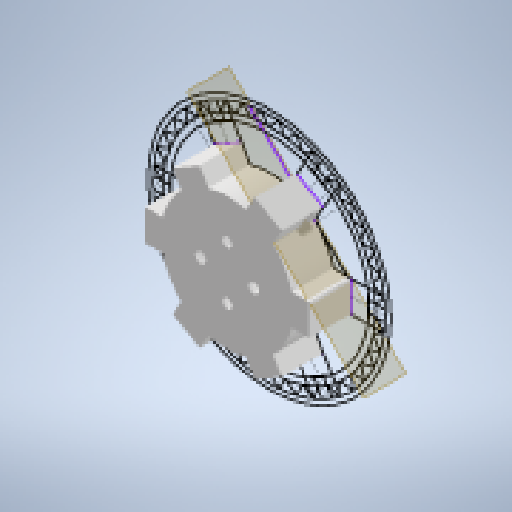
# Autodesk Inventor part: inside_part_wheel
Saved by Autodesk Inventor 2023 (Build 270158000, 158)
## iProperties
Created: 2026-02-22
Part Number: inside_part_wheel
Material: Типовые
Document SubType Name: Modeling
Designer: garin
Density: 1 g/cm^3
Appearance: По умолчанию
Author: garin
Autodesk Inventor part; units mm, degrees
note: some values were not read from the file. Chosen so that the rebuilt part matches the saved one: second side of "Выдавливание1".
ref_plane "YZ Plane" through (0, 0, 0) normal (1, 0, 0) x (0, 1, 0)
sketch "Эскиз1" plane through (0, 0, 0) normal (0, 0, 1) x (1, 0, 0)
  line L0 (0, 0) -> (34.5691, 5.4752) construction
  line L1 (0, 0) -> (35, 0) construction
  line L2 (0, 0) -> (34.5691, -5.4752) construction
  circle A0 centre (0, 0) radius 11.25
  circle A1 centre (0, 0) radius 15
  circle A2 centre (0, 0) radius 20
  circle A3 centre (0, 0) radius 30.0525
  circle A4 centre (0, 0) radius 32.0038
  circle A5 centre (0, 0) radius 35
  line L3 (0, 0) -> (17.5, -30.3109) construction
  circle A6 centre (0, -8) radius 1.5
  circle A7 centre (-8, 0) radius 1.5
  line L4 (0, 0) -> (-35, 0) construction
  line L5 (-29.6307, -4.693) -> (-19.4416, -4.693) construction
  line L6 (-29.6307, -4.693) -> (-19.4416, -4.693)
  line L7 (-29.6839, -4.693) -> (-29.6839, 4.693)
  line L8 (-19.4416, 4.693) -> (-34.6839, 4.693) construction
  line L9 (-19.4416, -4.693) -> (-34.6839, -4.693) construction
  line L10 (10.751, 28.0074) -> (5.6565, 19.1834) construction
  line L11 (5.6565, 19.1834) -> (13.2777, 32.3837) construction
  line L12 (-5.6565, 19.1834) -> (-13.2777, 32.3837) construction
  circle A8 centre (0, 8) radius 1.5
  line L13 (0, 0) -> (-17.5, 30.3109) construction
  line L14 (-5.6565, 19.1834) -> (-13.2777, 32.3837)
  line L15 (0, 0) -> (17.5, 30.3109) construction
  line L16 (0, 0) -> (-17.5, -30.3109) construction
  line L17 (5.6565, 19.1834) -> (13.2777, 32.3837)
  line L18 (13.3758, 26.5536) -> (16.0133, 31.1219)
  line L19 (16.3082, 24.8605) -> (18.9457, 29.4289)
  line L20 (18.9457, 29.4289) -> (17.4457, 26.8308) construction
  line L21 (29.6307, 4.693) -> (19.4416, 4.693)
  line L22 (18.8796, -23.3144) -> (13.7851, -14.4904) construction
  line L23 (13.7851, -14.4904) -> (21.4063, -27.6907) construction
  line L24 (29.6839, 4.693) -> (29.6839, 1.693)
  line L25 (29.6839, 4.693) -> (29.6839, -4.693)
  line L26 (29.6839, -4.693) -> (29.6839, -1.693) construction
  circle A9 centre (8, 0) radius 1.5
  line L27 (-18.8796, 23.3144) -> (-13.7851, 14.4904) construction
  line L28 (-13.7851, 14.4904) -> (-21.4063, 27.6907) construction
  line L29 (-18.8796, 23.3144) -> (-13.7851, 14.4904)
  line L30 (-13.7851, 14.4904) -> (-21.4063, 27.6907)
  line L31 (-18.9063, 23.3605) -> (-10.7777, 28.0536)
  line L32 (-16.3082, 24.8605) -> (-18.9457, 29.4289)
  line L33 (-13.3758, 26.5536) -> (-16.0133, 31.1219)
  line L34 (-13.7851, -14.4904) -> (-21.4063, -27.6907) construction
  line L35 (-10.751, -28.0074) -> (-5.6565, -19.1834) construction
  line L36 (-13.7851, -14.4904) -> (-21.4063, -27.6907)
  line L37 (-10.751, -28.0074) -> (-5.6565, -19.1834)
  line L38 (13.7851, 14.4904) -> (21.4063, 27.6907) construction
  line L39 (21.4063, 27.6907) -> (20.1674, 25.5449) construction
  line L40 (10.7777, 28.0536) -> (18.9063, 23.3605)
  line L41 (13.7851, 14.4904) -> (21.4063, 27.6907)
  line L42 (10.751, 28.0074) -> (5.6565, 19.1834)
  line L43 (0, 0) -> (21.2118, 27.8399) construction
  line L44 (0, 0) -> (8, 0) construction
  line L45 (0, 0) -> (0, 8) construction
  line L46 (-10.7777, -28.0536) -> (-18.9063, -23.3605)
  line L47 (-13.3758, -26.5536) -> (-16.0133, -31.1219)
  line L48 (-16.3082, -24.8605) -> (-18.9457, -29.4289)
  line L49 (-5.6565, -19.1834) -> (-13.2777, -32.3837) construction
  line L50 (5.6565, -19.1834) -> (13.2777, -32.3837) construction
  line L51 (-5.6565, -19.1834) -> (-13.2777, -32.3837)
  line L52 (18.8796, -23.3144) -> (13.7851, -14.4904)
  line L53 (5.6565, -19.1834) -> (13.2777, -32.3837)
  line L54 (16.3082, -24.8605) -> (18.9457, -29.4289)
  line L55 (13.7851, -14.4904) -> (21.4063, -27.6907)
  line L56 (13.3758, -26.5536) -> (16.0133, -31.1219)
  line L57 (18.9063, -23.3605) -> (10.7777, -28.0536)
  line L58 (27.6414, 16.1308) -> (28.831, 19.8437)
  line L59 (24.938, 20.0584) -> (28.831, 19.8437)
  line L60 (24.7499, 20.2901) -> (25.3388, 24.1443)
  line L61 (21.4607, 23.742) -> (25.3388, 24.1443)
  line L62 (17.4457, 26.8308) -> (21.2118, 27.8399)
  line L63 (21.2384, 23.9411) -> (21.2118, 27.8399)
  line L64 (-19.4416, 4.693) -> (-34.6839, 4.693)
  line L65 (-17.4453, 26.8311) -> (-21.2113, 27.8403)
  line L66 (-21.238, 23.9415) -> (-21.2113, 27.8403)
  line L67 (-21.4603, 23.7424) -> (-25.3384, 24.1447)
  line L68 (-24.7496, 20.2905) -> (-25.3384, 24.1447)
  line L69 (-24.9377, 20.0588) -> (-28.8307, 19.8442)
  line L70 (-27.6411, 16.1312) -> (-28.8307, 19.8442)
  line L71 (-27.7903, 15.8727) -> (-31.6007, 15.0465)
  line L72 (-29.8401, 11.5678) -> (-31.6007, 15.0465)
  line L73 (-29.9467, 11.289) -> (-33.5789, 9.8719)
  line L74 (-31.2916, 6.7145) -> (-33.5789, 9.8719)
  line L75 (-31.3528, 6.4224) -> (-34.716, 4.45)
  line L76 (-29.6839, -1.693) -> (-34.959, -1.693)
  line L77 (-19.4416, -4.693) -> (-34.6839, -4.693)
  line L78 (-29.6839, 1.693) -> (-34.959, 1.693)
  line L79 (-31.959, 1.693) -> (-34.716, 4.45)
  line L80 (-31.9591, -1.6925) -> (-34.716, -4.4494)
  line L81 (-31.3529, -6.4219) -> (-34.716, -4.4494)
  line L82 (-31.2917, -6.714) -> (-33.5791, -9.8714)
  line L83 (-29.9469, -11.2885) -> (-33.5791, -9.8714)
  line L84 (-29.8403, -11.5673) -> (-31.6009, -15.046)
  line L85 (-27.7906, -15.8723) -> (-31.6009, -15.046)
  line L86 (-24.938, -20.0584) -> (-28.831, -19.8437)
  line L87 (-27.6414, -16.1308) -> (-28.831, -19.8437)
  line L88 (-17.4457, -26.8308) -> (-21.2118, -27.8399)
  line L89 (-21.2384, -23.9411) -> (-21.2118, -27.8399)
  line L90 (-21.4607, -23.742) -> (-25.3388, -24.1443)
  line L91 (-24.7499, -20.2901) -> (-25.3388, -24.1443)
  line L92 (-14.5138, -28.5236) -> (-13.5047, -32.2897)
  line L93 (-10.1149, -30.3634) -> (-13.5047, -32.2897)
  line L94 (-9.8313, -30.4564) -> (-8.2407, -34.016)
  line L95 (-5.1973, -31.579) -> (-8.2407, -34.016)
  line L96 (-4.9026, -31.6261) -> (-2.7702, -34.8902)
  line L97 (-0.1495, -32.0035) -> (-2.7702, -34.8902)
  line L98 (0.149, -32.0035) -> (2.7697, -34.8902)
  line L99 (-14.5133, 28.5238) -> (-13.5042, 32.2899)
  line L100 (-10.1144, 30.3635) -> (-13.5042, 32.2899)
  line L101 (-9.8308, 30.4565) -> (-8.2401, 34.0162)
  line L102 (-5.1968, 31.5791) -> (-8.2401, 34.0162)
  line L103 (14.5138, 28.5236) -> (13.5047, 32.2897)
  line L104 (10.1149, 30.3634) -> (13.5047, 32.2897)
  line L105 (9.8313, 30.4564) -> (8.2407, 34.016)
  line L106 (5.1973, 31.579) -> (8.2407, 34.016)
  line L107 (4.9026, 31.6261) -> (2.7702, 34.8902)
  line L108 (0.1495, 32.0035) -> (2.7702, 34.8902)
  line L109 (-4.9021, 31.6262) -> (-2.7697, 34.8902)
  line L110 (-0.149, 32.0035) -> (-2.7697, 34.8902)
  line L111 (14.5133, -28.5238) -> (13.5042, -32.2899)
  line L112 (5.1968, -31.5791) -> (8.2401, -34.0162)
  line L113 (9.8308, -30.4565) -> (8.2401, -34.0162)
  line L114 (10.1144, -30.3635) -> (13.5042, -32.2899)
  line L115 (17.4453, -26.8311) -> (21.2113, -27.8403)
  line L116 (21.238, -23.9415) -> (21.2113, -27.8403)
  line L117 (4.9021, -31.6262) -> (2.7697, -34.8902)
  line L118 (19.4416, -4.693) -> (34.6839, -4.693)
  line L119 (29.6839, -1.693) -> (34.959, -1.693)
  line L120 (21.4603, -23.7424) -> (25.3384, -24.1447)
  line L121 (24.7496, -20.2905) -> (25.3384, -24.1447)
  line L122 (24.9377, -20.0588) -> (28.8307, -19.8442)
  line L123 (27.6411, -16.1312) -> (28.8307, -19.8442)
  line L124 (27.7903, -15.8727) -> (31.6007, -15.0465)
  line L125 (29.9467, -11.289) -> (33.5789, -9.8719)
  line L126 (31.2916, -6.7145) -> (33.5789, -9.8719)
  line L127 (31.3528, -6.4224) -> (34.716, -4.45)
  line L128 (31.959, -1.693) -> (34.716, -4.45)
  line L129 (29.8401, -11.5678) -> (31.6007, -15.0465)
  line L130 (34.5691, 5.4752) -> (29.6307, 4.693) construction
  line L131 (19.4416, 4.693) -> (34.6839, 4.693)
  line L132 (34.6839, 4.693) -> (29.6839, 4.693) construction
  line L133 (29.6839, 1.693) -> (34.959, 1.693)
  line L134 (29.8403, 11.5673) -> (31.6009, 15.046)
  line L135 (31.2917, 6.714) -> (33.5791, 9.8714)
  line L136 (31.9591, 1.6925) -> (34.716, 4.4494)
  line L137 (31.3529, 6.4219) -> (34.716, 4.4494)
  line L138 (29.9469, 11.2885) -> (33.5791, 9.8714)
  line L139 (27.7906, 15.8723) -> (31.6009, 15.046)
  circle A10 centre (0, 0) radius 36.5
  line L140 (0, 0) -> (-24.7487, 24.7487) construction
  line L141 (0, 0) -> (35, 0) construction
  line L142 (0, 0) -> (-24.6962, 0) construction
  line L143 (-24.6962, -4.693) -> (-24.6962, 4.693)
  line L144 (-8.2838, -23.734) -> (-16.4124, -19.041)
  line L145 (16.4124, -19.041) -> (8.2838, -23.734)
  line L146 (24.6962, 4.693) -> (24.6962, -4.693)
  line L147 (8.2838, 23.734) -> (16.4124, 19.041)
  line L148 (-16.4124, 19.041) -> (-8.2838, 23.734)
  line L149 (0, 0) -> (21.2503, 21.2503) construction
  line L150 (0, 0) -> (30.0525, 0) construction
  line L151 (14.1421, 14.1421) -> (23.5912, 4.693)
  line L152 (23.5912, 4.693) -> (-6.168, 34.4522)
  circle A11 centre (0, 15) radius 2.1
  circle A12 centre (0, -15) radius 2.1
  point P0 (0, 0)
  point P1 (18.9062, 23.3604)
  point P2 (18.9055, 23.3609)
  point P3 (10.7784, 28.0531)
  point P4 (-10.7784, 28.0531)
  point P5 (-18.9055, 23.3609)
  point P6 (-18.9062, 23.3604)
  point P7 (-29.6838, 4.693)
  point P8 (-29.6839, 4.6922)
  point P9 (-29.6839, -4.6922)
  point P10 (-18.9055, -23.3609)
  point P11 (-10.7784, -28.0531)
  point P12 (-10.7776, -28.0534)
  point P13 (10.7776, -28.0534)
  point P14 (10.7784, -28.0531)
  point P15 (18.9055, -23.3609)
  point P16 (29.6839, -4.6922)
  point P17 (29.6839, 4.6922)
  point P18 (29.6838, 4.693)
  point P19 (-29.6838, -4.693)
  point P20 (-18.9062, -23.3604)
  point P21 (18.9062, -23.3604)
  point P22 (29.6838, -4.693)
  point P23 (10.7776, 28.0534)
  point P24 (-10.7776, 28.0534)
  point P25 (-24.6962, 4.693)
  point P26 (24.6962, -4.693)
  dimension "d10" = 70
  dimension "d21" = 60.105
  dimension "d31" = 30
  dimension "d11" = 40
  dimension "d12" = 9
  dimension "d13" = 5
  dimension "d14" = 360
  dimension "d15" = 360
  dimension "d16" = 5
  dimension "d17" = 90
  dimension "d18" = 3
  dimension "d19" = 3
  dimension "d20" = 360
  dimension "d22" = 3
  dimension "d23" = 45
  dimension "d24" = 45.392
  dimension "d25" = 360
  dimension "d26" = 22.5
  dimension "d27" = 8
  dimension "d28" = 3
  dimension "d29" = 8
  dimension "d30" = 3
  dimension "d32" = 73
  dimension "d45" = 135
  dimension "d48" = 360
  dimension "d54" = 45
  dimension "d63" = 4.2
  constraints: 306 end point, 46 point on line, 10 coincident, 9 centre point, 7 symmetric about line, 4 horizontal, 4 perpendicular, 3 equal length, 2 point on circle, 1 tangent, 1 vertical, 1 vertical alignment, 417 other
  measures "d11" diameter of A2
  measures "d12" angle of L1 L0
  measures "d13" distance of L0.end L130.end
  measures "d16" distance of L132.start L24.start
  measures "d17" angle of L25 L132
  measures "d18" distance of L24.start L24.end
  measures "d19" distance of L25.end L119.start
  measures "d22" distance of L20.start L20.end
  measures "d23" angle of L62 L20
  measures "d26" diameter of A0
  measures "d27" distance of L44.start L45.end
  measures "d28" diameter of A8
  measures "d29" distance of L44.start L44.end
  measures "d30" diameter of A9
  measures "d32" diameter of A10
  measures "d45" angle of L141 L140
  measures "d54" angle of L150 L149
  measures "d63" diameter of A11
extrude "Выдавливание1" add sketch "Эскиз1" along normal blind 11.5 contours A1 A12 A11 | A11 A1 | A1 A11 | A12 A1 | A1 A12 | A2
extrude "Выдавливание4" add sketch "Эскиз1" along normal blind 1 from surface at 11.5 contours A0 | A1 A12 A11 | A11 A1 | A1 A11 | A12 A1 | A1 A12 | A2
ref_plane "РабПлоскость1" through (-24.7024, -23.7395, 10.5) normal (0, 0, 1) x (1, 0, 0)
ref_plane "РабПлоскость2" through (-24.7024, -23.7395, 9) normal (0, 0, -1) x (0, 1, 0)
extrude "Выдавливание7" add sketch "Эскиз1" along normal blind 12.5 contours A2 L21 L146 L118 | L52 L145 L53 A2 | A2 L17 L152 L41 | L152 L17 L147 L41 | L37 L144 L36 A2 | A2 L29 L148 L14 | L6 L143 L64 A2
ref_plane "РабПлоскость3" through (23.5912, 4.693, 0) normal (0.7071068, 0.7071068, 0) x (-0.7071068, 0.7071068, 0)
sketch "Эскиз2" plane through (23.5912, 4.693, 0) normal (0.7071068, 0.7071068, 0) x (-0.7071068, 0.7071068, 0)
  line L0 (13.363, 0) -> (13.363, 3.5)
  line L1 (13.8618, 0) -> (13.8618, 12.5) projected
  line L2 (13.363, 0) -> (16.863, 0) construction
  circle A0 centre (13.363, 3.5) radius 2
  dimension "d56" = 3.5
  dimension "d57" = 90
  dimension "d58" = 4
  constraints: 4 end point, 1 centre point, 1 coincident, 1 horizontal, 1 parallel, 1 perpendicular
  measures "d56" distance of L0.start L0.end
  measures "d57" angle of L2 L0
  measures "d58" diameter of A0
extrude "Выдавливание8" cut sketch "Эскиз2" along normal blind 5.1 and the other way blind 9
sketch "Эскиз3" plane through (0, 0, 0) normal (0, 0, -1) x (-1, 0, 0)
  point P0 (0, 0)
extrude "Выдавливание9" cut sketch "Эскиз1" along normal blind 6 contours A0 | A11 A1 | A1 A11 | A12 A1 | A1 A12 | A6 | A7 | A8 | A9
